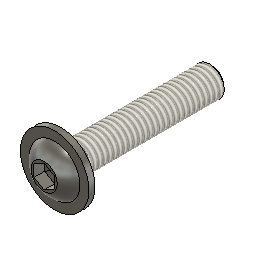
Smart Hoop_fusion_archive (Autodesk Fusion 360 archive; units mm, degrees)
design "Hexagon Socket Button Head Screw With Collar SFS-EN ISO 7380-2 - M6 x 30 Steel 4.6 Plain"
description: Hexagon Socket Button Head Screw With Collar SFS-EN ISO 7380-2 - M6 x 30
part number: SFS-EN ISO 7380-2 - M6 x 30 Steel 4.6 Plain
Autodesk Fusion 360 part; units mm, degrees
sketch "Sketch1" plane through (0, 0, 0) normal (0, 1, 0) x (1, 0, 0)
  line L0 (-3, 0) -> (-3, 30)
  line L1 (-3, 30) -> (0, 30)
  line L2 (0, 30) -> (0, -3.3)
  line L3 (0, -3.3) -> (-2.6, -3.3)
  arc A0 (-5, -1.2) -> (-2.6, -3.3) centre (0, 2.0929) ccw
  line L4 (-3, 0) -> (-6.8, 0)
  line L5 (-6.8, -1.2) -> (-5, -1.2)
  line L6 (-6.8, -1.2) -> (-6.8, 0)
  dimension "d9" = 6
  dimension "d66" = 10
  dimension "d98" = 5.2
  dimension "d106" = 30
  dimension "d114" = 13.6
  dimension "d117" = 1.2
  dimension "d120" = 3.3
  constraint perpendicular L0 L1
  constraint vertical L0
  constraint vertical L2
  constraint perpendicular L2 L3
  constraint coincident L2 A0.centre
  constraint perpendicular L0 L4
  constraint perpendicular L4 L6
  constraint horizontal L5
  constraint coincident origin L2
  constraint coincident origin L4
  measures "d106" distance of origin L1
  measures "d117" distance of L4 L5
  measures "d120" distance of L3 L4
revolve "Revolve1" add sketch "Sketch1" angle 360 about axis through (0, 0, -30) along (0, 0, 1)
ref_plane "WorkPlane1" through (0, 0, 3.3) normal (0, 0, 1) x (1, 0, 0)
sketch "Sketch6" plane through (0, 0, 3.3) normal (0, 0, 1) x (1, 0, 0)
  line L0 (0, -2.3094) -> (2, -1.1547)
  line L1 (2, -1.1547) -> (2, 1.1547)
  line L2 (2, 1.1547) -> (0, 2.3094)
  line L3 (0, 2.3094) -> (-2, 1.1547)
  line L4 (-2, 1.1547) -> (-2, -1.1547)
  line L5 (-2, -1.1547) -> (0, -2.3094)
  dimension "d127" = 4
  constraint vertical L1
  measures "d127" distance of L1 L4
extrude "Extrude1" cut sketch "Sketch6" against normal blind 2.08
extrude "Extrude2" cut 1 faces at (-0.6667, -0.3849, 1.22) along direction (0, 0, -1) blind 2.08 draft -85
thread "Thread5" "ISO Metric profile 6.0 M6x1 M6x1 6g" major diameter 5.884 minor diameter 4.7435 pitch 1 angle 60 resizes the face on face at (-2.9963, 0.1495, -20) from (0, 0, -3) to (0, 0, -30)
sketch "Sketch5" plane through (0, 0, 0) normal (0, 1, 0) x (1, 0, 0)
  line L0 (0, 30) -> (0, -3.3)
  line L1 (0, 30) -> (-3.06, 30)
  line L2 (-3.06, 30) -> (-3.06, 29.3865)
  line L3 (-3.06, 29.3865) -> (-2.3865, 30)
  dimension "d108" = 0.6135
  dimension "d109" = 2.3866
  dimension "d110" = 3.06
  constraint coincident L0.start L1.start
  constraint perpendicular L1 L2
  constraint coincident L1 L3.end
  measures "d108" distance of L1 L2.end
  measures "d109" distance of L0 L3.end
  measures "d110" distance of L0 L2
revolve "Revolve2" cut sketch "Sketch5" angle 360 about axis through (0, 0, -30) along (0, 0, 1)
fillet "Fillet6" radius 0.5 1 edges at (2.942, 0, 0)
equation "d9 = adsk_nomdia"
equation "adsk_nomlen = 30.00 mm"
equation "adsk_headh = 3.30 mm"
equation "adsk_headdia = 13.60 mm"
equation "adsk_nomdia = 6.00 mm"
equation "adsk_philwidth = 4.00 mm"
equation "d31 = -adsk_phildepth"
equation "adsk_phildepth = 2.08 mm"
equation "d66 = adsk_topdia"
equation "d71 = adsk_headh"
equation "d76 = -adsk_phildepth"
equation "adsk_thrlen = 27.00 mm"
equation "adsk_endpointdia = 4.7731 mm"
equation "adsk_startlen = 0.61345 mm"
equation "d98 = adsk_philwidth * 1.3"
equation "adsk_midfillet = 0.50 mm"
equation "d106 = adsk_nomlen"
equation "d108 = adsk_startlen"
equation "d109 = adsk_endpointdia / 2"
equation "d110 = adsk_nomdia * 0.51"
equation "adsk_flngheig = 1.20 mm"
equation "adsk_topdia = 10.00 mm"
equation "d114 = adsk_headdia"
equation "d117 = adsk_flngheig"
equation "d119 = adsk_midfillet"
equation "d120 = adsk_headh"
equation "d126 = min(adsk_thrlen; adsk_nomlen - adsk_midfillet - 0.001 mm)"
equation "d127 = adsk_philwidth"

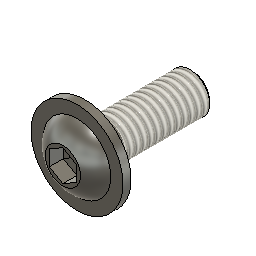
design "Hexagon Socket Button Head Screw With Collar SFS-EN ISO 7380-2 - M6 x 16 Steel 4.6 Plain"
description: Hexagon Socket Button Head Screw With Collar SFS-EN ISO 7380-2 - M6 x 16
part number: SFS-EN ISO 7380-2 - M6 x 16 Steel 4.6 Plain
Autodesk Fusion 360 part; units mm, degrees
sketch "Sketch1" plane through (0, 0, 0) normal (0, 1, 0) x (1, 0, 0)
  line L0 (-3, 0) -> (-3, 16)
  line L1 (-3, 16) -> (0, 16)
  line L2 (0, 16) -> (0, -3.3)
  line L3 (0, -3.3) -> (-2.6, -3.3)
  arc A0 (-5, -1.2) -> (-2.6, -3.3) centre (0, 2.0929) ccw
  line L4 (-3, 0) -> (-6.8, 0)
  line L5 (-6.8, -1.2) -> (-5, -1.2)
  line L6 (-6.8, -1.2) -> (-6.8, 0)
  dimension "d9" = 6
  dimension "d66" = 10
  dimension "d98" = 5.2
  dimension "d106" = 16
  dimension "d114" = 13.6
  dimension "d117" = 1.2
  dimension "d120" = 3.3
  constraint perpendicular L0 L1
  constraint vertical L0
  constraint vertical L2
  constraint perpendicular L2 L3
  constraint coincident L2 A0.centre
  constraint perpendicular L0 L4
  constraint perpendicular L4 L6
  constraint horizontal L5
  constraint coincident origin L2
  constraint coincident origin L4
  measures "d106" distance of origin L1
  measures "d117" distance of L4 L5
  measures "d120" distance of L3 L4
revolve "Revolve1" add sketch "Sketch1" angle 360 about axis through (0, 0, -16) along (0, 0, 1)
ref_plane "WorkPlane1" through (0, 0, 3.3) normal (0, 0, 1) x (1, 0, 0)
sketch "Sketch6" plane through (0, 0, 3.3) normal (0, 0, 1) x (1, 0, 0)
  line L0 (0, -2.3094) -> (2, -1.1547)
  line L1 (2, -1.1547) -> (2, 1.1547)
  line L2 (2, 1.1547) -> (0, 2.3094)
  line L3 (0, 2.3094) -> (-2, 1.1547)
  line L4 (-2, 1.1547) -> (-2, -1.1547)
  line L5 (-2, -1.1547) -> (0, -2.3094)
  dimension "d127" = 4
  constraint vertical L1
  measures "d127" distance of L1 L4
extrude "Extrude1" cut sketch "Sketch6" against normal blind 2.08
extrude "Extrude2" cut 1 faces at (-0.6667, -0.3849, 1.22) along direction (0, 0, -1) blind 2.08 draft -85
thread "Thread5" "ISO Metric profile 6.0 M6x1 M6x1 6g" major diameter 5.884 minor diameter 4.7435 pitch 1 angle 60 resizes the face on face at (-2.9963, 0.1495, -5.3333) from (0, 0, -3) to (0, 0, -16)
sketch "Sketch5" plane through (0, 0, 0) normal (0, 1, 0) x (1, 0, 0)
  line L0 (0, 16) -> (0, -3.3)
  line L1 (0, 16) -> (-3.06, 16)
  line L2 (-3.06, 16) -> (-3.06, 15.3866)
  line L3 (-3.06, 15.3866) -> (-2.3865, 16)
  dimension "d108" = 0.6135
  dimension "d109" = 2.3866
  dimension "d110" = 3.06
  constraint coincident L0.start L1.start
  constraint perpendicular L1 L2
  constraint coincident L1 L3.end
  measures "d108" distance of L1 L2.end
  measures "d109" distance of L0 L3.end
  measures "d110" distance of L0 L2
revolve "Revolve2" cut sketch "Sketch5" angle 360 about axis through (0, 0, -16) along (0, 0, 1)
fillet "Fillet6" radius 0.5 1 edges at (2.942, 0, 0)
equation "d9 = adsk_nomdia"
equation "adsk_nomlen = 16.00 mm"
equation "adsk_headh = 3.30 mm"
equation "adsk_headdia = 13.60 mm"
equation "adsk_nomdia = 6.00 mm"
equation "adsk_philwidth = 4.00 mm"
equation "d31 = -adsk_phildepth"
equation "adsk_phildepth = 2.08 mm"
equation "d66 = adsk_topdia"
equation "d71 = adsk_headh"
equation "d76 = -adsk_phildepth"
equation "adsk_thrlen = 13.00 mm"
equation "adsk_endpointdia = 4.7731 mm"
equation "adsk_startlen = 0.61345 mm"
equation "d98 = adsk_philwidth * 1.3"
equation "adsk_midfillet = 0.50 mm"
equation "d106 = adsk_nomlen"
equation "d108 = adsk_startlen"
equation "d109 = adsk_endpointdia / 2"
equation "d110 = adsk_nomdia * 0.51"
equation "adsk_flngheig = 1.20 mm"
equation "adsk_topdia = 10.00 mm"
equation "d114 = adsk_headdia"
equation "d117 = adsk_flngheig"
equation "d119 = adsk_midfillet"
equation "d120 = adsk_headh"
equation "d126 = min(adsk_thrlen; adsk_nomlen - adsk_midfillet - 0.001 mm)"
equation "d127 = adsk_philwidth"

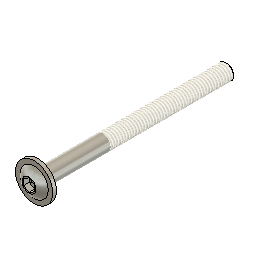
design "Hexagon Socket Button Head Screw With Collar SFS-EN ISO 7380-2 - M3 x 35 Steel 4.6 Plain"
description: Hexagon Socket Button Head Screw With Collar SFS-EN ISO 7380-2 - M3 x 35
part number: SFS-EN ISO 7380-2 - M3 x 35 Steel 4.6 Plain
Autodesk Fusion 360 part; units mm, degrees
sketch "Sketch1" plane through (0, 0, 0) normal (0, 1, 0) x (1, 0, 0)
  line L0 (-1.5, 0) -> (-1.5, 35)
  line L1 (-1.5, 35) -> (0, 35)
  line L2 (0, 35) -> (0, -1.65)
  line L3 (0, -1.65) -> (-1.3, -1.65)
  arc A0 (-2.6, -0.7) -> (-1.3, -1.65) centre (0, 1.4934) ccw
  line L4 (-1.5, 0) -> (-3.45, 0)
  line L5 (-3.45, -0.7) -> (-2.6, -0.7)
  line L6 (-3.45, -0.7) -> (-3.45, 0)
  dimension "d9" = 3
  dimension "d66" = 5.2
  dimension "d98" = 2.6
  dimension "d106" = 35
  dimension "d114" = 6.9
  dimension "d117" = 0.7
  dimension "d120" = 1.65
  constraint perpendicular L0 L1
  constraint vertical L0
  constraint vertical L2
  constraint perpendicular L2 L3
  constraint coincident L2 A0.centre
  constraint perpendicular L0 L4
  constraint perpendicular L4 L6
  constraint horizontal L5
  constraint coincident origin L2
  constraint coincident origin L4
  measures "d106" distance of origin L1
  measures "d117" distance of L4 L5
  measures "d120" distance of L3 L4
revolve "Revolve1" add sketch "Sketch1" angle 360 about axis through (0, 0, -35) along (0, 0, 1)
ref_plane "WorkPlane1" through (0, 0, 1.65) normal (0, 0, 1) x (1, 0, 0)
sketch "Sketch6" plane through (0, 0, 1.65) normal (0, 0, 1) x (1, 0, 0)
  line L0 (0, -1.1547) -> (1, -0.5774)
  line L1 (1, -0.5774) -> (1, 0.5774)
  line L2 (1, 0.5774) -> (0, 1.1547)
  line L3 (0, 1.1547) -> (-1, 0.5774)
  line L4 (-1, 0.5774) -> (-1, -0.5774)
  line L5 (-1, -0.5774) -> (0, -1.1547)
  dimension "d127" = 2
  constraint vertical L1
  measures "d127" distance of L1 L4
extrude "Extrude1" cut sketch "Sketch6" against normal blind 1.04
extrude "Extrude2" cut 1 faces at (-0.3333, -0.1925, 0.61) along direction (0, 0, -1) blind 1.04 draft -85
thread "Thread5" "ISO Metric profile 3.0 M3x0.5 M3x0.5 6g" major diameter 2.927 minor diameter 2.3555 pitch 0.5 angle 60 resizes the face on face at (-1.4981, 0.0748, -11.6667) from (0, 0, -12) to (0, 0, -35)
sketch "Sketch5" plane through (0, 0, 0) normal (0, 1, 0) x (1, 0, 0)
  line L0 (0, 35) -> (0, -1.65)
  line L1 (0, 35) -> (-1.53, 35)
  line L2 (-1.53, 35) -> (-1.53, 34.6933)
  line L3 (-1.53, 34.6933) -> (-1.1933, 35)
  dimension "d108" = 0.3067
  dimension "d109" = 1.1933
  dimension "d110" = 1.53
  constraint coincident L0.start L1.start
  constraint perpendicular L1 L2
  constraint coincident L1 L3.end
  measures "d108" distance of L1 L2.end
  measures "d109" distance of L0 L3.end
  measures "d110" distance of L0 L2
revolve "Revolve2" cut sketch "Sketch5" angle 360 about axis through (0, 0, -35) along (0, 0, 1)
fillet "Fillet6" radius 0.3333 1 edges at (1.4635, 0, 0)
equation "d9 = adsk_nomdia"
equation "adsk_nomlen = 35.00 mm"
equation "adsk_headh = 1.65 mm"
equation "adsk_headdia = 6.90 mm"
equation "adsk_nomdia = 3.00 mm"
equation "adsk_philwidth = 2.00 mm"
equation "d31 = -adsk_phildepth"
equation "adsk_phildepth = 1.04 mm"
equation "d66 = adsk_topdia"
equation "d71 = adsk_headh"
equation "d76 = -adsk_phildepth"
equation "adsk_thrlen = 23.00 mm"
equation "adsk_endpointdia = 2.38655 mm"
equation "adsk_startlen = 0.306725 mm"
equation "d98 = adsk_philwidth * 1.3"
equation "adsk_midfillet = 0.3333 mm"
equation "d106 = adsk_nomlen"
equation "d108 = adsk_startlen"
equation "d109 = adsk_endpointdia / 2"
equation "d110 = adsk_nomdia * 0.51"
equation "adsk_flngheig = 0.70 mm"
equation "adsk_topdia = 5.20 mm"
equation "d114 = adsk_headdia"
equation "d117 = adsk_flngheig"
equation "d119 = adsk_midfillet"
equation "d120 = adsk_headh"
equation "d126 = min(adsk_thrlen; adsk_nomlen - adsk_midfillet - 0.001 mm)"
equation "d127 = adsk_philwidth"

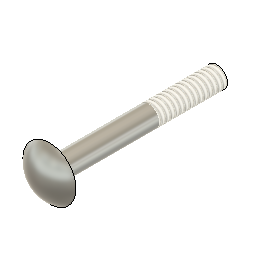
design "Round Head Fin Neck Bolt ASME B18.5 - I10-24 UNC x 1 1/2 Steel Grade 2 Plain"
description: Round Head Fin Neck Bolt ASME B18.5 - I10-24 UNC x 1 1/2
part number: RHFNB ASME B18.5 - I10-24 UNC x 1 1/2 Steel Grade 2 Plain
Autodesk Fusion 360 part; units mm, degrees
sketch "Sketch1" plane through (0, 0, 0) normal (0, 1, 0) x (1, 0, 0)
  line L0 (-2.413, 0) -> (-2.413, 38.1)
  line L1 (-2.413, 38.1) -> (0, 38.1)
  line L2 (0, 38.1) -> (0, -2.8956)
  line L3 (-2.413, 0) -> (-5.9563, 0)
  arc A0 (-5.9563, 0) -> (0, -2.8956) centre (0, 4.6783) ccw
  dimension "d9" = 4.826
  dimension "d66" = 11.9126
  dimension "d116" = 2.8956
  dimension "d117" = 38.1
  constraint perpendicular L0 L1
  constraint perpendicular L0 L3
  constraint coincident origin L3
  constraint vertical L0
  constraint vertical L2
  constraint coincident L2.end A0.end
  constraint coincident L2 A0.centre
  constraint coincident origin L2
  constraint coincident L3.end A0.start
  measures "d116" distance of L2.end L3
  measures "d117" distance of origin L1
revolve "Revolve1" add sketch "Sketch1" angle 360 about axis through (0, 0, -38.1) along (0, 0, 1)
fillet "Fillet4" radius 0.7874 1 edges at (-2.2497, 0.8726, 0)
sketch "Sketch9" plane through (0, 0, 0) normal (0, 0, 1) x (1, 0, 0)
  line L0 (0, 5.0165) -> (-2.413, 0)
  line L1 (-2.413, 0) -> (0, -5.0165)
  line L2 (0, -5.0165) -> (2.413, 0)
  line L3 (2.413, 0) -> (0, 5.0165)
  line L4 (-2.413, 0) -> (2.413, 0) construction
  line L5 (0, 0) -> (0, -5.0165) construction
  point P0 (-2.413, 0)
  dimension "d120" = 5.0165
  dimension "d124" = 2.413
  constraint vertical L0.start L5.start
  constraint horizontal P0 L2.end
  constraint vertical L0.start L1.end
  constraint horizontal L2.end L5.start
  constraint coincident P0 L0.end
  constraint coincident L5.start origin
  constraint parallel L1 L3
  measures "d120" distance of L1.end L4
  measures "d124" distance of L2.end L5
extrude "Extrude5" add sketch "Sketch9" against normal blind 4.9162 draft -35
thread "Thread2" "ANSI Unified Screw Threads 0.19(#10) 10-24 UNC 10-24 UNC 2A" major diameter 4.7092 minor diameter 3.5408 pitch 1.0583 angle 60 resizes the face on face at (-0.7038, -2.3081, -25.6625) from (0, 0, -22.225) to (0, 0, -38.1)
sketch "Sketch5" plane through (0, 0, 0) normal (0, 1, 0) x (1, 0, 0)
  line L0 (-2.4613, 38.1) -> (-2.4613, 37.4508)
  line L1 (-2.4613, 37.4508) -> (-1.4516, 38.1)
  line L2 (0, 38.1) -> (0, -2.8956)
  line L3 (-2.4613, 38.1) -> (0, 38.1)
  line L4 (0, 38.1) -> (0, 0) construction
  dimension "d121" = 1.4516
  dimension "d122" = 2.4613
  dimension "d123" = 0.6492
  constraint coincident L2.start L3.end
  constraint perpendicular L2 L3
  constraint coincident L1.end L3
  constraint perpendicular L0 L3
  constraint coincident L4.end origin
  measures "d121" distance of L1.end L4
  measures "d122" distance of L0 L2.start
  measures "d123" distance of L0.end L3
revolve "Revolve2" cut sketch "Sketch5" angle 360 about axis through (0, 0, -38.1) along (0, 0, 1)
equation "d9 = adsk_nomdia"
equation "d66 = adsk_headdia"
equation "adsk_nomlen = 1.50 in"
equation "adsk_headh = 0.114 in"
equation "adsk_headdia = 0.469 in"
equation "adsk_nomdia = 0.19 in"
equation "adsk_thrlen = 0.625 in"
equation "d91 = min(adsk_thrlen; adsk_nomlen - ( adsk_wafin - adsk_nomdia ) * 0.33)"
equation "adsk_endpointdia = 0.1143 in"
equation "adsk_startlen = 0.025561 in"
equation "adsk_wafin = 0.395 in"
equation "d110 = -adsk_wafin * 0.49"
equation "adsk_midfillet = 0.031 in"
equation "d115 = adsk_midfillet"
equation "d116 = adsk_headh"
equation "d117 = adsk_nomlen"
equation "d120 = adsk_wafin / 2"
equation "d121 = adsk_endpointdia / 2"
equation "d122 = adsk_nomdia * 0.51"
equation "d123 = adsk_startlen"
equation "d124 = ( min(adsk_wafin / 2; adsk_nomdia) ) / 2"
